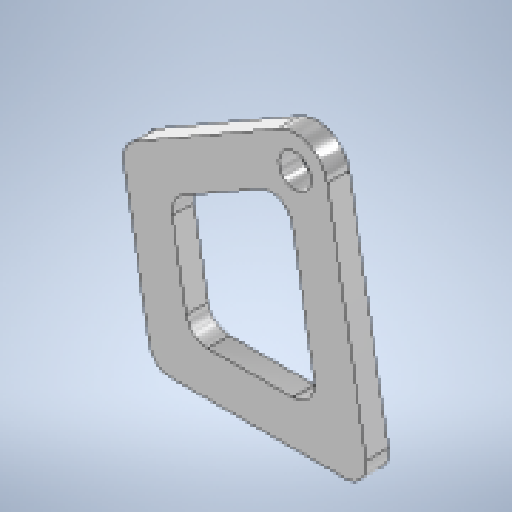
# Autodesk Inventor part: Uprights
Saved by Autodesk Inventor 2023.2 (Build 272271000, 271)
## iProperties
Created: 2024-01-11
Part Number: Uprights
Material: UHMW, White
Document SubType Name: Modeling
Designer: Nathan Cai
Mass: 15.8619 g
Surface Area: 82.8248 cm^2
Volume: 16.8743 cm^3
Density: 0.94 g/cm^3
Appearance: Smooth - White
Author: Nathan Cai
Autodesk Inventor part; units mm, degrees
ref_plane "YZ Plane" through (0, 0, 0) normal (1, 0, 0) x (0, 1, 0)
ref_plane "XZ Plane" through (0, 0, 0) normal (0, 1, 0) x (-1, 0, 0)
ref_plane "XY Plane" through (0, 0, 0) normal (0, 0, 1) x (1, 0, 0)
sketch "Sketch2" plane through (0, 0, 0) normal (0, 0, 1) x (1, 0, 0)
  circle A0 centre (0, 0) radius 4.7625
  circle A1 centre (0, 0) radius 9.525
  line L0 (-41.275, -69.85) -> (21.9884, -69.85)
  line L1 (-41.275, -69.85) -> (-50.3999, -18.0999)
  line L2 (-50.3999, -18.0999) -> (-4.7625, 8.2489)
  line L3 (9.3803, 1.654) -> (21.9884, -69.85)
  line L4 (-1.5674, -9.3952) -> (6.8531, -57.15)
  line L5 (6.8531, -57.15) -> (-29.0064, -57.15)
  line L6 (-29.0064, -57.15) -> (-34.8856, -23.8074)
  line L7 (-34.8856, -23.8074) -> (-6.1896, -7.2398)
  line L8 (-41.275, -69.85) -> (-140.0337, -69.85)
  line L9 (-50.3999, -18.0999) -> (-140.0337, -69.85)
  line L10 (-45.8375, -43.9749) -> (-31.767, -41.4939) construction
  line L11 (-34.0215, -51.5634) -> (-37.3295, -32.8028) construction
  line L12 (-37.3295, -32.8028) -> (-43.583, -33.9055) construction
  line L13 (-43.583, -33.9055) -> (-40.275, -52.6661) construction
  line L14 (-40.275, -52.6661) -> (-34.0215, -51.5634) construction
  line L15 (-34.0215, -51.5634) -> (-43.583, -33.9055) construction
  line L16 (-37.3295, -32.8028) -> (-40.275, -52.6661) construction
  circle A2 centre (-43.583, -33.9055) radius 2
  circle A3 centre (-40.275, -52.6661) radius 2
  circle A4 centre (-35.6755, -42.1831) radius 2
  point P0 (-38.8022, -42.7344)
  dimension "d6" = 9.525
  dimension "d7" = 19.05
  dimension "d14" = 69.85
  dimension "d15" = 100
  dimension "d16" = 41.275
  dimension "d17" = 110
  dimension "d18" = 12.7
  dimension "d19" = 12.7
  dimension "d20" = 14.2875
  dimension "d24" = 19.05
  dimension "d25" = 6.35
  dimension "d26" = 4
  dimension "d27" = 4
  dimension "d28" = 4
  dimension "d29" = 12.7
  constraints: 35 end point, 5 centre point, 5 midpoint, 5 parallel, 4 coincident, 4 point on circle, 2 horizontal, 2 perpendicular, 2 tangent, 1 collinear, 1 point on line
  measures "d6" diameter of A0
  measures "d7" diameter of A1
  measures "d14" distance from line of L0 A1.centre
  measures "d15" angle of L0 L1
  measures "d16" horizontal distance of A0.centre L0.start
  measures "d17" angle of L2 L1
  measures "d18" distance between parallel lines of L3 L4
  measures "d19" distance between parallel lines of L2 L7
  measures "d20" distance between parallel lines of L1 L6
  measures "d24" distance of L11.start L11.end
  measures "d25" distance of L12.end L11.end
  measures "d26" diameter of A2
  measures "d27" diameter of A3
  measures "d28" diameter of A4
  measures "d29" distance between parallel lines of L0 L5
extrude "Extrusion2" add sketch "Sketch2" along normal blind 6.35 contours A1 | A1 L3 L0 L1 L2 L7 L6 L5 L4
fillet "Fillet1" radius 6.35 8 edges at (21.9884, -69.85, 3.175) (6.8531, -57.15, 3.175) (-41.275, -69.85, 3.175) (-29.0064, -57.15, 3.175) (-34.8856, -23.8074, 3.175) (-50.3999, -18.0999, 3.175) (-6.1896, -7.2398, 3.175) (-1.5674, -9.3952, 3.175)
equation "\"d18\" = d19"
equation "\"d29\" = d19"
body "Solid2"
